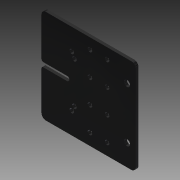
# Autodesk Inventor part: S2_Zplate
Saved by Autodesk Inventor 2013 SP2 (Build 170200200, 200)
## iProperties
Created: 2013-02-23
Part Number: S2_Zplate
Material: Steel, Mild
Document SubType Name: Modeling
Designer: Edward
Density: 7.86 g/cm^3
Mass: 310.643 g
Surface Area: 256.499 cm^2
Volume: 39.522 cm^3
Description: Z-axis spindle mount plate
Vendor: custom
Stock Number: SM_Z3
Author: Edward
Autodesk Inventor part; units mm, degrees
ref_plane "YZ Plane" through (0, 0, 0) normal (1, 0, 0) x (0, 1, 0)
ref_plane "XZ Plane" through (0, 0, 0) normal (0, 1, 0) x (-1, 0, 0)
ref_plane "XY Plane" through (0, 0, 0) normal (0, 0, 1) x (1, 0, 0)
sketch "Sketch1" plane through (0, 0, 0) normal (0, 0, 1) x (1, 0, 0)
  line L0 (-55, 55) -> (55, 55)
  line L1 (55, 55) -> (55, -55)
  line L2 (55, -55) -> (-55, -55)
  line L3 (-55, -55) -> (-55, 55)
  point P0 (0, 0)
  dimension "d0" = 110
  dimension "d1" = 110
  dimension "d2" = 55
  dimension "d3" = 55
  constraints: 8 end point, 2 parallel, 1 horizontal, 1 perpendicular
  measures "d0" distance of L1.end L2.end
  measures "d1" distance of L0.end L1.end
  measures "d2" distance from line of point (0, 0) L3
  measures "d3" distance from line of L0 point (0, 0)
extrude "Extrusion1" add sketch "Sketch1" along normal blind 3.4163
sketch "Sketch2" plane through (0, 0, 3.4163) normal (0, 0, 1) x (1, 0, 0)
  line L0 (55, 55) -> (-55, 55) projected
  circle A0 centre (45, 30) radius 3.57
  circle A1 centre (45, -30) radius 3.57
  circle A2 centre (-19.6, -30) radius 2.625
  circle A3 centre (-19.6, 30) radius 2.625
  circle A4 centre (-16.5, 24) radius 2.625
  circle A5 centre (-16.5, -24) radius 2.625
  line L1 (-55, -55) -> (55, -55) projected
  line L2 (55, -55) -> (55, 55) projected
  point P0 (0, 0)
  dimension "d6" = 7.14
  dimension "d7" = 7.14
  dimension "d8" = 5.25
  dimension "d9" = 5.25
  dimension "d10" = 60
  dimension "d11" = 25
  dimension "d12" = 64.6
  dimension "d13" = 64.6
  dimension "d14" = 60
  dimension "d16" = 25
  dimension "d20" = 5.25
  dimension "d21" = 5.25
  dimension "d22" = 71.5
  dimension "d23" = 31
  dimension "d24" = 31
  dimension "d25" = 71.5
  dimension "d27" = 10
  dimension "d28" = 10
  constraints: 6 centre point
  measures "d6" diameter of A0
  measures "d7" diameter of A1
  measures "d8" diameter of A2
  measures "d9" diameter of A3
  measures "d10" distance of A1.centre A0.centre
  measures "d11" distance from line of L0 A0.centre
  measures "d12" distance of A3.centre A0.centre
  measures "d13" distance of A2.centre A1.centre
  measures "d14" distance of A3.centre A2.centre
  measures "d16" distance from line of L0 A3.centre
  measures "d20" diameter of A4
  measures "d21" diameter of A5
  measures "d22" distance from line of L2 A4.centre
  measures "d23" distance from line of L0 A4.centre
  measures "d24" distance from line of L1 A5.centre
  measures "d25" distance from line of L2 A5.centre
  measures "d27" distance from line of L2 A0.centre
  measures "d28" distance from line of L2 A1.centre
extrude "Extrusion2" cut sketch "Sketch2" against normal through all
sketch "Sketch3" plane through (0, 0, 3.4163) normal (0, 0, 1) x (1, 0, 0)
  line L0 (55, 55) -> (-55, 55) projected
  arc A0 (-25, -2.625) -> (-25, 2.625) centre (-25, 0) ccw
  line L1 (-55, 55) -> (-55, -55) projected
  line L2 (-55, 2.625) -> (-25, 2.625)
  line L3 (-25, -2.625) -> (-55, -2.625)
  point P0 (0, 0)
  dimension "d30" = 5.25
  dimension "d33" = 55
  dimension "d38" = 30
  dimension "d39" = 30
  constraints: 4 end point, 2 point on circle, 2 point on line, 2 tangent, 1 centre point, 1 perpendicular
  measures "d30" diameter of A0
  measures "d33" distance from line of L0 A0.centre
  measures "d38" distance of L2.start L2.end
  measures "d39" distance of L3.start L3.end
extrude "Extrusion3" cut sketch "Sketch3" against normal through all
fillet "Fillet2" radius 5 4 edges at (-55, 55, 1.7082) (-55, -55, 1.7082) (55, 55, 1.7082) (55, -55, 1.7082)
sketch "Sketch4" plane through (0, 0, 3.4163) normal (0, 0, 1) x (1, 0, 0)
  line L0 (50, 55) -> (-50, 55) projected
  circle A0 centre (1.7, 42.5) radius 2.625
  point P0 (0, 0)
  dimension "d40" = 5.25
  dimension "d50" = 12.5
  constraints: 1 centre point
  measures "d40" diameter of A0
  measures "d50" distance from line of L0 A0.centre
extrude "Extrusion4" cut sketch "Sketch4" against normal through all
fillet "Fillet3" radius 2 2 edges at (-55, 2.625, 1.7082) (-55, -2.625, 1.7082)
pattern_linear "Rectangular Pattern1" count 2 spacing 20 along (1, 0, 0) count 4 spacing 28 along (0, -1, 0) of "Extrusion4"
equation "\"d2\" = 0.5 * d0"
equation "\"d3\" = 0.5 * d1"
equation "\"d13\" = d12"
equation "\"d14\" = d10"
equation "\"d16\" = d11"
equation "\"d24\" = d23"
equation "\"d25\" = d22"
equation "\"d39\" = d38"
body "Solid1"
